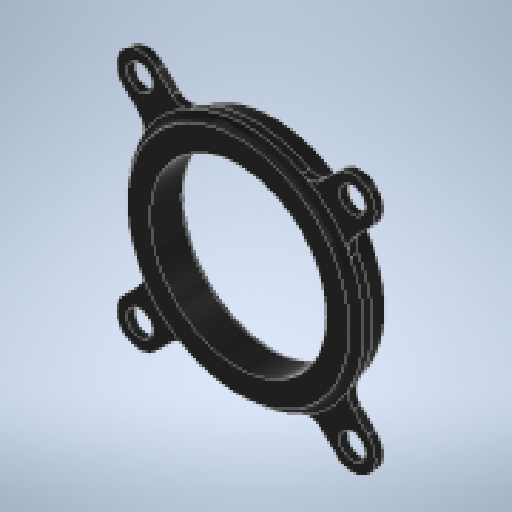
# Autodesk Inventor part: servohorn_support_forR0
Saved by Autodesk Inventor 2024.3 (Build 283343010, 343A)
## iProperties
Created: 2025-06-29
Part Number: servohorn_support_forR0
Material: 一般
Document SubType Name: Modeling
Designer: kshau
Density: 1 g/cm^3
Appearance: 滑らか - 黒
Author: kshau
Autodesk Inventor part; units mm, degrees
ref_plane "YZ Plane" through (0, 0, 0) normal (1, 0, 0) x (0, 1, 0)
ref_plane "XZ Plane" through (0, 0, 0) normal (0, 1, 0) x (-1, 0, 0)
ref_plane "XY Plane" through (0, 0, 0) normal (0, 0, 1) x (1, 0, 0)
sketch "スケッチ1" plane through (0, 0, 0) normal (0, 0, 1) x (1, 0, 0)
  circle A0 centre (0, 0) radius 19
  line L0 (0, 0) -> (0, 19)
  line L1 (0, 0) -> (13.435, 13.435)
  circle A1 centre (13.435, 13.435) radius 2.9
  circle A2 centre (-13.435, 13.435) radius 2.9
  circle A3 centre (-13.435, -13.435) radius 2.9
  circle A4 centre (13.435, -13.435) radius 2.9
  circle A5 centre (0, 0) radius 14.9
  line L2 (15.4856, -11.3844) -> (-11.3844, 15.4856)
  line L3 (-15.4856, 11.3844) -> (11.3844, -15.4856)
  line L4 (-15.4856, -11.3844) -> (11.3844, 15.4856)
  line L5 (15.4856, 11.3844) -> (-11.3844, -15.4856)
  point P0 (-11.2339, 15.3232)
  point P1 (-15.3232, 11.2339)
  point P2 (-15.3282, 11.227)
  point P3 (-12.385, 8.2838)
  point P4 (-12.385, -8.2838)
  point P5 (-15.3282, -11.227)
  point P6 (-15.3232, -11.2339)
  point P7 (-11.2339, -15.3232)
  point P8 (-11.227, -15.3282)
  point P9 (-8.2838, -12.385)
  point P10 (8.2838, -12.385)
  point P11 (11.227, -15.3282)
  point P12 (11.2339, -15.3232)
  point P13 (15.3232, -11.2339)
  point P14 (15.3282, -11.227)
  point P15 (12.385, -8.2838)
  point P16 (12.385, 8.2838)
  point P17 (15.3282, 11.227)
  point P18 (15.3232, 11.2339)
  point P19 (11.2339, 15.3232)
  point P20 (11.227, 15.3282)
  point P21 (8.2838, 12.385)
  point P22 (-8.2838, 12.385)
  point P23 (-11.227, 15.3282)
  dimension "d0" = 38
  dimension "d1" = 45
  dimension "d2" = 5.8
  dimension "d5" = 360
  dimension "d7" = 29.8
  constraints: 12 end point, 10 point on circle, 7 tangent, 6 centre point, 3 coincident, 1 perpendicular, 1 vertical, 9 other
  measures "d0" diameter of A0
  measures "d1" angle of L0 L1
  measures "d2" diameter of A1
  measures "d7" diameter of A5
extrude "押し出し1" add sketch "スケッチ1" along normal blind 1 contours L5 A5 L1 A1 A0 | A0 A4 L3 A5 L2 | A1 L1 A0 | A0 A1 | L5 L2 L1 A5 | A5 L2 L5 | A4 A0 | A0 A4 | A5 L3 L5 L2 | L1 A1 A0 | L1 A5 L4 A0 A1 | L1 L2 L4 A5 | L5 L3 L4 L0 L1 L2 | A5 L5 L3 | L1 L0 L2 | L4 L0 A5 | L5 A5 L4 L3 | L5 A0 A3 L4 A5 | L2 A5 L0 | L4 L3 A5 L2 | L4 A5 L3 | A5 L3 A0 A2 L2 | A3 A0 | A0 A3 | A2 A0 | A0 A2
sketch "スケッチ2" plane through (0, 0, 1) normal (0, 0, 1) x (1, 0, 0)
  circle A0 centre (0, 0) radius 14
  dimension "d10" = 28
  constraints: 1 centre point, 1 coincident
  measures "d10" diameter of A0
extrude "押し出し2" add sketch "スケッチ2" along normal blind 1
sketch "スケッチ3" plane through (0, 0, 0) normal (0, 0, -1) x (-1, 0, 0)
  circle A0 centre (0, 0) radius 14
  dimension "d13" = 28
  constraints: 1 centre point, 1 coincident
  measures "d13" diameter of A0
extrude "押し出し3" add sketch "スケッチ3" along normal blind 2.5
sketch "スケッチ4" plane through (0, 0, -2.5) normal (0, 0, -1) x (-1, 0, 0)
  circle A0 centre (0, 0) radius 11.1
  dimension "d16" = 22.2
  constraints: 1 centre point, 1 coincident
  measures "d16" diameter of A0
extrude "押し出し4" cut sketch "スケッチ4" against normal blind 6
sketch "スケッチ5" plane through (0, 0, -1) normal (0, 0, -1) x (-1, 0, 0)
  circle A0 centre (0, 0) radius 11
  dimension "d19" = 22
  constraints: 1 centre point, 1 coincident
  measures "d19" diameter of A0
extrude "押し出し5" [suppressed]
fillet "フィレット1" radius 1 1 edges at (-14, 0, 1)
sketch "スケッチ6" plane through (0, 0, 0) normal (0, 0, -1) x (-1, 0, 0)
  arc A0 (-15.3232, -11.2339) -> (-11.2339, -15.3232) centre (-13.435, -13.435) ccw projected
  arc A1 (11.2339, -15.3232) -> (15.3232, -11.2339) centre (13.435, -13.435) ccw projected
  arc A2 (15.3232, 11.2339) -> (11.2339, 15.3232) centre (13.435, 13.435) ccw projected
  arc A3 (-11.2339, 15.3232) -> (-15.3232, 11.2339) centre (-13.435, 13.435) ccw projected
  point P0 (0, 0)
  constraints: 4 coincident
hole "穴1" at (13.435, -13.435, 0) at (-13.435, -13.435, 0) at (-13.435, 13.435, 0) at (13.435, 13.435, 0) direction (0, 0, 1) diameter 3.2 end through all
fillet "フィレット2" radius 2 8 edges at (12.385, 8.2838, 0.5) (12.385, -8.2838, 0.5) (8.2838, -12.385, 0.5) (-8.2838, -12.385, 0.5) (-12.385, -8.2838, 0.5) (-8.2838, 12.385, 0.5) (-12.385, 8.2838, 0.5) (8.2838, 12.385, 0.5)
fillet "フィレット3" radius 0.5 1 edges at (14, 0, 0)
fillet "フィレット4" radius 0.5 1 edges at (11.1, 0, -2.5)
